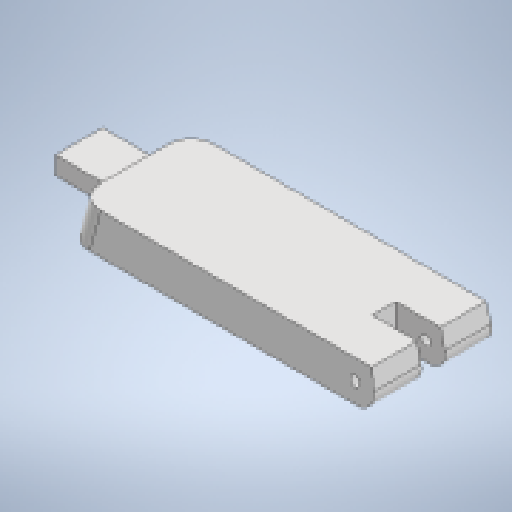
# Autodesk Inventor part: ArcherT4U_USB
Saved by Autodesk Inventor 2025.1 (Build 291241000, 241)
## iProperties
Created: 2026-04-16
Part Number: ArcherT4U_USB
Material: Generic
Document SubType Name: Modeling
Designer: User
Density: 1 g/cm^3
Appearance: Default
Author: User
Autodesk Inventor part; units mm, degrees
ref_plane "YZ Plane" through (0, 0, 0) normal (1, 0, 0) x (0, 1, 0)
sketch "Sketch1" plane through (0, 0, 0) normal (0, 1, 0) x (-1, 0, 0)
  line L0 (11.8992, 6.1446) -> (-67.1008, 6.1446)
  line L1 (-67.1008, 6.1446) -> (-67.1008, -24.4554)
  line L2 (-67.1008, -24.4554) -> (11.8992, -24.4554)
  line L3 (11.8992, -24.4554) -> (11.8992, 6.1446)
  point P0 (0, 0)
  dimension "d0" = 79
  dimension "d1" = 30.6
  constraints: 8 end point, 2 parallel, 1 horizontal, 1 perpendicular
  measures "d0" distance of L2.end L1.end
  measures "d1" distance of L1.end L0.end
extrude "Extrusion1" add sketch "Sketch1" along normal blind 9.51
sketch "Sketch3" plane through (-11.8992, 0, -24.4554) normal (-1, 0, 0) x (0, 0, 1)
  line L0 (0, 9.51) -> (30.6, 9.51) projected
  line L1 (15.3, 9.51) -> (0.75, 9.51)
  line L2 (30.6, 9.51) -> (0, 9.51) projected
  line L3 (0.75, 9.51) -> (29.85, 9.51)
  line L4 (30.6, 0) -> (30.6, 9.51) projected
  line L5 (0, 0) -> (0, 9.51) projected
  line L6 (30.6, 0) -> (0, 0) projected
  line L7 (30.6, 0) -> (29.85, 9.51)
  line L8 (0, 0) -> (0.75, 9.51)
  point P0 (24.4554, 0)
  dimension "d4" = 14.55
  dimension "d5" = 29.1
  constraints: 8 end point, 2 point on line, 1 midpoint
  measures "d4" distance of L1.start L1.end
  measures "d5" distance of L1.end L3.end
extrude "Extrusion2" cut sketch "Sketch3" against normal through all contours L0 L8 L5 | L7 L0 L4
ref_plane "Work Plane1" through (67.1008, 0, -24.4554) normal (0, 0, 1) x (-1, 0, 0)
sketch "Sketch5" plane through (67.1008, 0, -24.4554) normal (0, 0, 1) x (-1, 0, 0)
  line L0 (0, -9.51) -> (79, -9.51) projected
  line L1 (79, -9.51) -> (79, 0) projected
  line L2 (0, 0) -> (0, -9.51) projected
  line L3 (79, -9.51) -> (0, -9.51) projected
  line L4 (39.5, -9.51) -> (77, -9.51)
  line L5 (77, -9.51) -> (79, 0)
  line L6 (79, 0) -> (79, -9.51) projected
  line L7 (79, -9.51) -> (79, 0)
  line L8 (39.5, -9.51) -> (2, -9.51)
  line L9 (0, -9.51) -> (0, 0) projected
  line L10 (2, -9.51) -> (0, 0)
  line L11 (0, 0) -> (0, -9.51)
  line L12 (0, -9.51) -> (2, -9.51)
  point P0 (67.1008, 0)
  dimension "d11" = 37.5
  dimension "d12" = 37.5
  constraints: 14 end point, 3 collinear, 2 point on line, 1 midpoint
  measures "d11" distance of L4.start L4.end
  measures "d12" distance of L4.start L8.end
extrude "Extrusion3" cut sketch "Sketch5" along normal through all
ref_plane "Work Plane2" through (-11.8992, 0, -24.4554) normal (1, 0, 0) x (0, 0, 1)
sketch "Sketch7" plane through (-11.8992, 0, -24.4554) normal (1, 0, 0) x (0, 0, 1)
  line L0 (0, 0) -> (30.6, 0) projected
  line L1 (0.75, -9.51) -> (29.85, -9.51) projected
  line L2 (29.85, -9.51) -> (30.6, 0) projected
  line L3 (0, 0) -> (0.75, -9.51) projected
  line L4 (15.3, 0) -> (15.3, -9.51)
  line L5 (28.0015, -7.51) -> (2.5985, -7.51)
  line L6 (2.5985, -7.51) -> (2.1639, -2)
  line L7 (2.1639, -2) -> (28.4361, -2)
  line L8 (28.4361, -2) -> (28.0015, -7.51)
  line L9 (27.3541, -3) -> (3.2459, -3)
  line L10 (3.2459, -3) -> (3.5227, -6.51)
  line L11 (3.5227, -6.51) -> (27.0773, -6.51)
  line L12 (27.0773, -6.51) -> (27.3541, -3)
  line L13 (15.3, -3) -> (15.3, -7.51)
  line L14 (21.3, -3) -> (9.3, -3)
  line L15 (9.3, -3) -> (9.3, -7.51)
  line L16 (9.3, -7.51) -> (21.3, -7.51)
  line L17 (21.3, -7.51) -> (21.3, -3)
  line L18 (21.3, -3) -> (9.3, -7.51) construction
  line L19 (9.3, -3) -> (21.3, -7.51) construction
  point P0 (24.4554, 0)
  point P1 (15.3, -5.255)
  dimension "d16" = 2
  dimension "d17" = 3
  dimension "d18" = 12
  constraints: 32 end point, 7 midpoint, 2 parallel, 1 horizontal, 1 perpendicular, 1 point on line, 6 other
  measures "d16" distance between parallel lines of L1 L5
  measures "d17" distance between parallel lines of L0 L9
  measures "d18" distance of L16.end L15.end
extrude "Extrusion4" add sketch "Sketch7" along normal blind 10 contours L9 L17 L11 L4 | L4 L11 L15 L9 | L5 L15 L11 L4 | L4 L11 L17 L5
sketch "Sketch8" plane through (-11.8992, 0, -24.4554) normal (-1, 0, 0) x (0, 0, 1)
  line L0 (9.3, 7.51) -> (21.3, 7.51) projected
  line L1 (9.3, 3) -> (9.3, 7.51) projected
  line L2 (21.3, 3) -> (9.3, 3) projected
  line L3 (21.3, 7.51) -> (21.3, 3) projected
  point P0 (24.4554, 0)
extrude "Extrusion5" add sketch "Sketch8" along normal blind 12
sketch "Sketch9" plane through (67.1008, 0, -24.4554) normal (0, 0, 1) x (-1, 0, 0)
  line L0 (0, 0) -> (79, 0) projected
  line L1 (2, -9.51) -> (77, -9.51) projected
  line L2 (0, -4.755) -> (79, -4.755)
  line L3 (2, -9.51) -> (0, 0) projected
  line L4 (4.9287, 0) -> (79, 0)
  line L5 (1.0143, -4.8232) -> (2, -9.51)
  arc A0 (4.9287, 0) -> (1.0143, -4.8232) centre (4.9287, -4) ccw
  point P0 (67.1008, 0)
  point P1 (4.9287, 0)
  dimension "d23" = 9.51
  dimension "d24" = 4.755
  dimension "d25" = 4
  constraints: 6 end point, 2 point on circle, 2 point on line, 2 tangent, 1 centre point, 1 collinear, 1 horizontal, 1 parallel
  measures "d23" distance between parallel lines of L1 L0
  measures "d24" distance between parallel lines of L0 L2
  measures "d25" radius of A0
extrude "Extrusion6" cut sketch "Sketch9" along normal through all
sketch "Sketch10" plane through (67.1008, 0, -24.4554) normal (0, 0, 1) x (-1, 0, 0)
  line L0 (4.9287, 0) -> (79, 0) projected
  line L1 (2, -9.51) -> (77, -9.51) projected
  line L2 (4.9287, -4.755) -> (79, -4.755)
  line L3 (2, -9.51) -> (1.0143, -4.8232) projected
  circle A0 centre (5.859, -4.755) radius 4.755
  circle A1 centre (5.859, -4.755) radius 1.25
  point P0 (67.1008, 0)
  dimension "d28" = 9.51
  dimension "d29" = 4.755
  dimension "d31" = 2.5
  constraints: 2 centre point, 2 end point, 2 tangent, 1 coincident, 1 parallel
  measures "d28" distance between parallel lines of L1 L0
  measures "d29" distance between parallel lines of L0 L2
  measures "d31" diameter of A1
extrude "Extrusion7" cut sketch "Sketch10" along normal through all contours A1
sketch "Sketch11" plane through (0, 0, 0) normal (0, -1, 0) x (1, 0, 0)
  line L0 (-11.8992, 6.1446) -> (62.1721, 6.1446) projected
  line L1 (62.1721, -24.4554) -> (-11.8992, -24.4554) projected
  line L2 (-11.8992, -6.1554) -> (62.1721, -6.1554)
  line L3 (62.1721, -12.1554) -> (-11.8992, -12.1554)
  line L4 (25.1364, -6.1554) -> (66.0864, -6.1554)
  line L5 (66.0864, 5.7642) -> (66.0864, -24.075) projected
  line L6 (25.1364, -12.1554) -> (66.0864, -12.1554)
  line L7 (65.1008, 5.3946) -> (65.1008, -23.7054) projected
  line L8 (66.0864, -6.1554) -> (53.6864, -6.1554)
  line L9 (53.6864, -6.1554) -> (53.6864, -12.1554)
  line L10 (66.1721, 5.8291) -> (66.1721, -24.1399) projected
  line L11 (66.0864, -6.1554) -> (66.1721, -6.1554)
  line L12 (66.0864, -12.1554) -> (66.1721, -12.1554)
  point P0 (0, 0)
  dimension "d34" = 12.3
  dimension "d35" = 12.3
  dimension "d36" = 12.4
  constraints: 16 end point, 5 point on line, 4 perpendicular, 2 midpoint, 2 parallel, 1 horizontal
  measures "d34" distance between parallel lines of L0 L2
  measures "d35" distance between parallel lines of L1 L3
  measures "d36" distance of L4.end L8.end
extrude "Extrusion8" cut sketch "Sketch11" against normal through all
fillet "Fillet1" radius 6 2 edges at (-10.8992, 4.755, 5.7696) (-10.8992, 4.755, -24.0804)
ref_plane "Work Plane3" through (65.1008, 9.51, -16.8054) normal (0.205803, -0.9785934, 0) x (0, 0, -1)
body "Solid1"
